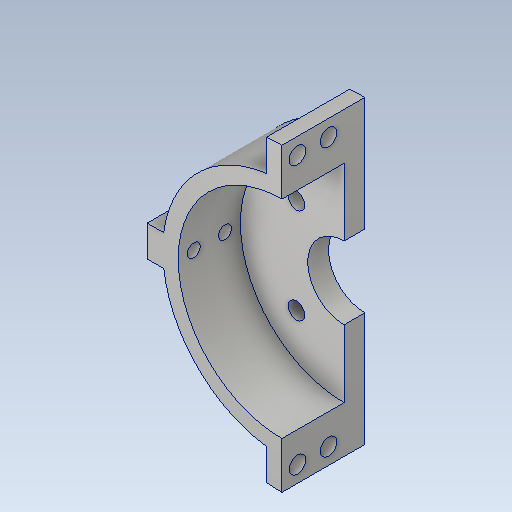
# Autodesk Inventor part: 조인트4링크2고정부
Saved by Autodesk Inventor 2020 (Build 240168000, 168)
## iProperties
Created: 2021-07-09
Part Number: 조인트4링크2고정부
Material: 알루미늄 6061
Document SubType Name: Modeling
Designer: user
Density: 2.7 g/cm^3
Appearance: 알루미늄 - 평지
Mass: 16.4675 g
Surface Area: 44.8155 cm^2
Volume: 6.09906 cm^3
Author: user
Autodesk Inventor part; units mm, degrees
ref_plane "YZ Plane" through (0, 0, 0) normal (1, 0, 0) x (0, 1, 0)
ref_plane "XZ Plane" through (0, 0, 0) normal (0, 1, 0) x (-1, 0, 0)
ref_plane "XY Plane" through (0, 0, 0) normal (0, 0, 1) x (1, 0, 0)
sketch "스케치1" plane through (0, 0, 0) normal (0, 0, 1) x (1, 0, 0)
  arc A0 (0, 7) -> (0, -7) centre (0, 0) ccw
  arc A1 (0, 23) -> (0, -23) centre (0, 0) ccw
  line L0 (0, 0) -> (0, 23)
  line L1 (0, 0) -> (0, -23)
  dimension "d0" = 14
  dimension "d1" = 46
  constraints: 4 end point, 4 point on circle, 3 point on line, 2 centre point, 2 coincident, 1 vertical
  measures "d0" diameter of A0
  measures "d1" diameter of A1
extrude "돌출1" add sketch "스케치1" along normal blind 4 contours A0 L1 A1 L0
sketch "스케치2" plane through (0, 0, 4) normal (0, 0, 1) x (1, 0, 0)
  arc A0 (0, 20) -> (0, -20) centre (0, 0) ccw
  arc A1 (0, 23) -> (0, -23) centre (0, 0) ccw
  line L0 (0, 20) -> (0, 29)
  line L1 (0, 0) -> (0, -29)
  arc A2 (-3, -28.8444) -> (0, -29) centre (0, 0) ccw
  arc A3 (0, 29) -> (-3, 28.8444) centre (0, 0) ccw
  line L2 (-3, 28.8444) -> (-3, 19.7737)
  line L3 (-3, -19.7737) -> (-3, -22.8035)
  line L4 (-3, -28.8444) -> (-3, -19.7737)
  line L5 (-3, 19.7737) -> (-3, 28.8444)
  line L6 (-3, 22.8035) -> (-3, 19.7737)
  line L7 (-3, -19.7737) -> (-3, -28.8444)
  line L8 (0, -29) -> (0, -20)
  line L9 (0, 20) -> (0, 29)
  line L10 (0, 29) -> (0, 20)
  line L11 (0, -20) -> (0, -29)
  dimension "d4" = 40
  dimension "d5" = 46
  dimension "d6" = 29
  dimension "d7" = 29
  constraints: 24 end point, 12 point on circle, 8 parallel, 4 centre point, 3 coincident, 3 point on line, 2 collinear, 2 vertical
  measures "d4" diameter of A0
  measures "d5" diameter of A1
  measures "d6" distance of L1.start L0.end
  measures "d7" distance of L1.start L1.end
extrude "돌출2" add sketch "스케치2" along normal blind 12
sketch "스케치3" plane through (-3, -28.8444, 4) normal (-1, 0, 0) x (0, 0, 1)
  line L0 (0, 51.6479) -> (12, 51.6479) projected
  line L1 (12, 57.6888) -> (12, 51.6479) projected
  line L2 (0, 57.6888) -> (12, 57.6888) projected
  line L3 (0, 57.6888) -> (0, 51.6479) projected
  line L4 (12, 6.0409) -> (0, 6.0409) projected
  line L5 (0, 6.0409) -> (0, 0) projected
  line L6 (0, 0) -> (12, 0) projected
  line L7 (12, 6.0409) -> (12, 0) projected
  circle A0 centre (9, 3) radius 1.6
  circle A1 centre (3, 3) radius 1.6
  circle A2 centre (9, 54.6888) radius 1.6
  circle A3 centre (3, 54.6888) radius 1.6
  point P0 (-4, 28.8444)
  dimension "d16" = 3.2
  dimension "d17" = 3.2
  dimension "d18" = 3.2
  dimension "d19" = 3.2
  dimension "d20" = 3
  dimension "d21" = 3
  dimension "d22" = 3
  dimension "d23" = 3
  dimension "d24" = 3
  dimension "d25" = 3
  dimension "d26" = 3
  dimension "d27" = 3
  constraints: 4 centre point
  measures "d16" diameter of A0
  measures "d17" diameter of A1
  measures "d18" diameter of A2
  measures "d19" diameter of A3
  measures "d20" distance from line of L1 A2.centre
  measures "d21" distance from line of L3 A3.centre
  measures "d22" distance from line of L2 A2.centre
  measures "d23" distance from line of L2 A3.centre
  measures "d24" distance from line of L6 A1.centre
  measures "d25" distance from line of A1.centre L5
  measures "d26" distance from line of L6 A0.centre
  measures "d27" distance from line of L7 A0.centre
extrude "돌출3" cut sketch "스케치3" against normal up to surface (3 mm away) contours A0 | A1 | A2 | A3
sketch "스케치5" plane through (0, 0, 16) normal (0, 0, 1) x (1, 0, 0)
  circle A0 centre (0, 0) radius 23
  arc A1 (-3, 22.8035) -> (-3, -22.8035) centre (0, 0) ccw projected
  line L0 (-23, 0) -> (-26, 0)
  line L1 (-23, 0) -> (-20, 0) construction
  line L2 (-26, 0) -> (-26, -3)
  line L3 (-26, -3) -> (-22.8035, -3)
  line L4 (-26, 0) -> (-26, 3)
  line L5 (-26, 0) -> (-23, 0) construction
  line L6 (-26, 3) -> (-22.8035, 3)
  dimension "d36" = 46
  dimension "d37" = 3
  dimension "d38" = 180
  dimension "d39" = 3
  dimension "d40" = 90
  dimension "d41" = 90
  dimension "d42" = 3
  dimension "d43" = 90
  constraints: 14 end point, 3 horizontal, 3 point on circle, 2 equal length, 1 centre point, 1 coincident, 1 perpendicular, 1 vertical
  measures "d36" diameter of A0
  measures "d37" distance of L0.start L0.end
  measures "d38" angle of L0 L1
  measures "d39" distance of L0.end L2.end
  measures "d40" angle of L2 L0
  measures "d41" angle of L3 L2
  measures "d42" distance of L0.end L4.end
  measures "d43" angle of L5 L4
extrude "돌출5" add sketch "스케치5" against normal blind 16 contours A0 L0 L4 L6 | L3 L2 L0 A0
sketch "스케치6" plane through (-26, -3, 16) normal (-1, 0, 0) x (0, 0, 1)
  line L0 (0, 6) -> (0, 0) projected
  line L1 (0, 6) -> (-16, 6) projected
  line L2 (-16, 0) -> (-16, 6) projected
  line L3 (0, 0) -> (-16, 0) projected
  circle A0 centre (-3, 3) radius 1.25
  circle A1 centre (-9, 3) radius 1.25
  point P0 (-16, 3)
  dimension "d46" = 2.5
  dimension "d47" = 2.5
  dimension "d48" = 3
  dimension "d49" = 7
  dimension "d50" = 3
  dimension "d51" = 3
  constraints: 2 centre point
  measures "d46" diameter of A0
  measures "d47" diameter of A1
  measures "d48" distance from line of L0 A0.centre
  measures "d49" distance from line of L2 A1.centre
  measures "d50" distance from line of L1 A1.centre
  measures "d51" distance from line of L1 A0.centre
extrude "돌출6" cut sketch "스케치6" against normal blind 8 contours A0 | A1
sketch "스케치7" plane through (0, 0, 4) normal (0, 0, 1) x (1, 0, 0)
  circle A0 centre (0, 0) radius 13
  line L0 (0, 0) -> (-9.1924, 9.1924)
  line L1 (0, 0) -> (13, 0) construction
  line L2 (0, 0) -> (-9.1924, -9.1924)
  line L3 (0, 0) -> (13, 0) construction
  circle A1 centre (-9.1924, 9.1924) radius 1.6
  circle A2 centre (-9.1924, -9.1924) radius 1.6
  dimension "d54" = 26
  dimension "d55" = 135
  dimension "d56" = 135
  dimension "d57" = 3.2
  dimension "d58" = 3.2
  constraints: 8 end point, 3 centre point, 3 coincident, 2 equal length, 2 horizontal, 2 point on circle
  measures "d54" diameter of A0
  measures "d55" angle of L1 L0
  measures "d56" angle of L2 L3
  measures "d57" diameter of A1
  measures "d58" diameter of A2
extrude "돌출7" cut sketch "스케치7" against normal up to surface (4 mm away) contours A1 L0 A0 | A0 A1 | A2 A0 | A0 L2 A2 | L0 A1 A0 | A0 A2 L2
sketch "스케치8" plane through (0, 0, 0) normal (0, 0, -1) x (-1, 0, 0)
  arc A0 (3, 22.8035) -> (0, 23) centre (0, 0) ccw projected
  line L0 (3, 28.8444) -> (3, 22.8035) projected
  arc A1 (3, 28.8444) -> (0, 29) centre (0, 0) ccw projected
  line L1 (0, 23) -> (0, 29) projected
  arc A2 (0, -23) -> (3, -22.8035) centre (0, 0) ccw projected
  line L2 (0, -29) -> (0, -23) projected
  arc A3 (0, -29) -> (3, -28.8444) centre (0, 0) ccw projected
  line L3 (3, -22.8035) -> (3, -28.8444) projected
extrude "돌출8" add sketch "스케치8" against normal blind 4
